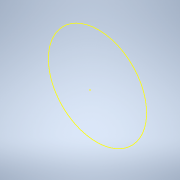
# Autodesk Inventor part: Ручной привод
Saved by Autodesk Inventor 2020 (Build 240168000, 168)
## iProperties
Created: 2020-12-08
Part Number: Ручной привод
Material: Типовые
Document SubType Name: Modeling
Designer: User
Density: 1 g/cm^3
Appearance: По умолчанию
Author: User
Autodesk Inventor part; units mm, degrees
ref_plane "YZ Plane" through (0, 0, 0) normal (1, 0, 0) x (0, 1, 0)
ref_plane "XZ Plane" through (0, 0, 0) normal (0, 1, 0) x (-1, 0, 0)
ref_plane "XY Plane" through (0, 0, 0) normal (0, 0, 1) x (1, 0, 0)
sketch "Эскиз1" plane through (0, 0, 0) normal (0, 0, 1) x (1, 0, 0)
  circle A0 centre (0, 0) radius 22
  line L0 (-4, 4) -> (4, 4)
  line L1 (4, 4) -> (4, -4)
  line L2 (4, -4) -> (-4, -4)
  line L3 (-4, -4) -> (-4, 4)
  line L4 (-4, 4) -> (4, -4) construction
  line L5 (4, 4) -> (-4, -4) construction
  circle A1 centre (0, 13.3333) radius 2
  circle A2 centre (-13.3333, 0) radius 2
  circle A3 centre (0, -13.3333) radius 2
  circle A4 centre (13.3333, 0) radius 2
  dimension "d0" = 44
  dimension "d1" = 8
  dimension "d2" = 8
  dimension "d3" = 4
  dimension "d5" = 13.3333
  dimension "d6" = 0
  dimension "d9" = 360
  constraints: 12 end point, 5 centre point, 2 midpoint, 2 parallel, 1 coincident, 1 horizontal, 1 perpendicular, 9 other
  measures "d0" diameter of A0
  measures "d1" distance of L1.end L2.end
  measures "d2" distance of L0.end L1.end
  measures "d3" diameter of A1
  measures "d5" distance of point (0, 0) A1.centre
  measures "d6" horizontal distance of point (0, 0) A1.centre
extrude "Выдавливание1" add sketch "Эскиз1" against normal blind 16 contours A0 | A1 | A2 | A3 | A4
hole "Отверстие1" at (13.3333, 0, 0) direction (0, 0, -1) diameter 4 end through all clearance for "с потайной головкой ГОСТ 12876-67" size "M4" standard "ГОСТ"
hole "Отверстие2" at (-13.3333, 0, 0) direction (0, 0, -1) diameter 4 end through all clearance for "с потайной головкой ГОСТ 12876-67" size "M4" standard "ГОСТ"
chamfer "Фаска1" distance 2 angle 45 1 edges at (-22, 0, -16)
ref_plane "РабПлоскость1" through (109, -4, 0) normal (-1, 0, 0) x (0, 0, 1)
sketch "Эскиз2" plane through (4, -4, 0) normal (-1, 0, 0) x (0, 0, 1)
  line L0 (0, -18) -> (0, 26) projected
  line L1 (-14, 26) -> (-14, -18) projected
  line L2 (-14, -18) -> (0, -18)
  line L3 (-14, 26) -> (0, 26)
  constraints: 4 end point, 2 horizontal
sketch "Эскиз3" plane through (109, -4, 0) normal (-1, 0, 0) x (0, 0, 1)
  line L0 (0, -18) -> (0, 26) construction
  line L1 (-14, 26) -> (-14, -18) construction
  line L2 (0, -6.5) -> (-14, -6.5)
  line L3 (-14, -6.5) -> (-14, 14.5)
  line L4 (-14, 14.5) -> (0, 14.5)
  line L5 (0, 14.5) -> (0, -6.5)
  point P0 (0, 4)
  point P1 (0, 4)
  dimension "d53" = 21
  dimension "d54" = 14
  constraints: 8 end point, 2 collinear, 2 midpoint, 2 parallel, 1 horizontal, 1 perpendicular
  measures "d53" distance between parallel lines of L2 L4
  measures "d54" distance between parallel lines of L1 L0
sketch "Эскиз4" plane through (0, 0, 0) normal (0, 0, 1) x (1, 0, 0)
  circle A0 centre (0, 0) radius 22 construction
  line L0 (0, -22) -> (0, -4)
  arc A1 (0, 22) -> (109, 10.5) centre (90.7698, 360.0249) ccw
  arc A2 (109, -10.5) -> (0, -22) centre (90.7698, -360.0249) ccw
  line L1 (109, -10.5) -> (109, 10.5)
  circle A3 centre (13.3333, 0) radius 2 projected
  line L2 (4, 4) -> (4, -4) projected
  line L3 (-4, 4) -> (4, 4) projected
  line L4 (4, -4) -> (-4, -4) projected
  line L5 (0, -4) -> (0, 4) construction
  line L6 (0, 4) -> (0, 22)
  line L7 (0, -43.0669) -> (0, 43.0669) construction
  arc A4 (109, -10.5) -> (109, 10.5) centre (109, 0) ccw
  point P0 (109, 10.5)
  point P1 (109, -10.5)
  dimension "d55" = 350
  dimension "d56" = 350
  constraints: 10 end point, 8 point on circle, 5 vertical, 4 midpoint, 3 centre point, 1 coincident, 1 point on line
  measures "d55" radius of A1
  measures "d56" radius of A2
extrude "Выдавливание2" add sketch "Эскиз4" against normal blind 14
equation "\"d53\" = 1.5 * d54"
equation "\"d56\" = d55"
